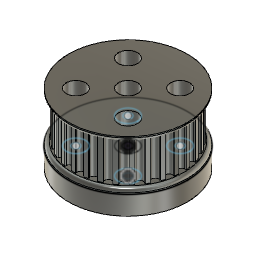
M5_Pulley_t30 v3 (Autodesk Fusion 360 design; units mm, degrees)
Autodesk Fusion 360 part; units mm, degrees
sketch "Sketch1" plane through (0, 0, 0) normal (0, 0, 1) x (1, 0, 0)
  circle A0 centre (0, 0) radius 25
  circle A1 centre (0, 0) radius 4
  circle A2 centre (0, 0) radius 1.75
  circle A3 centre (10.9602, -10.9602) radius 1.5
  circle A4 centre (10.9602, -10.9602) radius 4
  circle A5 centre (10.9602, 10.9602) radius 4
  circle A6 centre (10.9602, 10.9602) radius 1.5
  circle A7 centre (-10.9602, 10.9602) radius 4
  circle A8 centre (-10.9602, 10.9602) radius 1.5
  circle A9 centre (-10.9602, -10.9602) radius 4
  circle A10 centre (-10.9602, -10.9602) radius 1.5
  point P0 (10.9602, -10.9602)
  dimension "d1" = 50
  dimension "d2" = 8
  dimension "d3" = 3.5
  dimension "d25" = 360
  constraint coincident A0.centre A1.centre
  constraint concentric A0 A2
  constraint coincident P0 A3.centre
  measures "d1" diameter of A0
  measures "d2" diameter of A1
  measures "d3" diameter of A2
sketch "Sketch3" plane through (0, 0, 0) normal (0, 0, 1) x (1, 0, 0)
  line L0 (22.3838, 1.4892) -> (22.9524, 1.5279)
  line L1 (22.9524, -1.5279) -> (22.3838, -1.4892)
  arc A0 (22.3838, 1.4892) -> (22.3838, -1.4892) centre (22.4332, 0) ccw
  line L2 (21.585, 6.1105) -> (22.1332, 6.2666)
  arc A1 (21.585, 6.1105) -> (22.2042, 3.1972) centre (21.943, 4.6641) ccw
  line L3 (22.7685, 3.2776) -> (22.2042, 3.1972)
  line L4 (19.8429, 10.4647) -> (20.3467, 10.7314)
  arc A2 (19.8429, 10.4647) -> (21.0543, 7.7439) centre (20.4938, 9.1244) ccw
  line L5 (21.5895, 7.9398) -> (21.0543, 7.7439)
  line L6 (17.2335, 14.3616) -> (17.6709, 14.7272)
  arc A3 (17.2335, 14.3616) -> (18.9842, 11.9521) centre (18.1489, 13.1859) ccw
  line L7 (19.467, 12.255) -> (18.9842, 11.9521)
  line L8 (13.871, 17.6308) -> (14.2228, 18.0793)
  arc A4 (13.871, 17.6308) -> (16.0843, 15.6379) centre (15.0108, 16.6711) ccw
  line L9 (16.4936, 16.0347) -> (16.0843, 15.6379)
  line L10 (9.9022, 20.1295) -> (10.1531, 20.6413)
  arc A5 (9.9022, 20.1295) -> (12.4815, 18.6403) centre (11.2166, 19.4278) ccw
  line L11 (12.7994, 19.1135) -> (12.4815, 18.6403)
  line L12 (5.5007, 21.7484) -> (5.6396, 22.3012)
  arc A6 (5.5007, 21.7484) -> (8.3333, 20.828) centre (6.9323, 21.3353) ccw
  line L13 (8.5458, 21.3569) -> (8.3333, 20.828)
  line L14 (0.8587, 22.4168) -> (0.8797, 22.9864)
  arc A7 (0.8587, 22.4168) -> (3.8208, 22.1055) centre (2.3449, 22.3103) ccw
  line L15 (3.9187, 22.667) -> (3.8208, 22.1055)
  line L16 (-3.8208, 22.1055) -> (-3.9187, 22.667)
  arc A8 (-3.8208, 22.1055) -> (-0.8587, 22.4168) centre (-2.3449, 22.3103) ccw
  line L17 (-0.8797, 22.9864) -> (-0.8587, 22.4168)
  line L18 (-8.3333, 20.828) -> (-8.5458, 21.3569)
  arc A9 (-8.3333, 20.828) -> (-5.5007, 21.7484) centre (-6.9323, 21.3353) ccw
  line L19 (-5.6396, 22.3012) -> (-5.5007, 21.7484)
  line L20 (-12.4815, 18.6403) -> (-12.7994, 19.1135)
  arc A10 (-12.4815, 18.6403) -> (-9.9022, 20.1295) centre (-11.2166, 19.4278) ccw
  line L21 (-10.1531, 20.6413) -> (-9.9022, 20.1295)
  line L22 (-16.0843, 15.6379) -> (-16.4936, 16.0347)
  arc A11 (-16.0843, 15.6379) -> (-13.871, 17.6308) centre (-15.0108, 16.6711) ccw
  line L23 (-14.2228, 18.0793) -> (-13.871, 17.6308)
  line L24 (-18.9842, 11.9521) -> (-19.467, 12.255)
  arc A12 (-18.9842, 11.9521) -> (-17.2335, 14.3616) centre (-18.1489, 13.1859) ccw
  line L25 (-17.6709, 14.7272) -> (-17.2335, 14.3616)
  line L26 (-21.0543, 7.7439) -> (-21.5895, 7.9398)
  arc A13 (-21.0543, 7.7439) -> (-19.8429, 10.4647) centre (-20.4938, 9.1244) ccw
  line L27 (-20.3467, 10.7314) -> (-19.8429, 10.4647)
  line L28 (-22.2042, 3.1972) -> (-22.7685, 3.2776)
  arc A14 (-22.2042, 3.1972) -> (-21.585, 6.1105) centre (-21.943, 4.6641) ccw
  line L29 (-22.1332, 6.2666) -> (-21.585, 6.1105)
  line L30 (-22.3838, -1.4892) -> (-22.9524, -1.5279)
  arc A15 (-22.3838, -1.4892) -> (-22.3838, 1.4892) centre (-22.4332, 0) ccw
  line L31 (-22.9524, 1.5279) -> (-22.3838, 1.4892)
  line L32 (-21.585, -6.1105) -> (-22.1332, -6.2666)
  arc A16 (-21.585, -6.1105) -> (-22.2042, -3.1972) centre (-21.943, -4.6641) ccw
  line L33 (-22.7685, -3.2776) -> (-22.2042, -3.1972)
  line L34 (-19.8429, -10.4647) -> (-20.3467, -10.7314)
  arc A17 (-19.8429, -10.4647) -> (-21.0543, -7.7439) centre (-20.4938, -9.1244) ccw
  line L35 (-21.5895, -7.9398) -> (-21.0543, -7.7439)
  line L36 (-17.2335, -14.3616) -> (-17.6709, -14.7272)
  arc A18 (-17.2335, -14.3616) -> (-18.9842, -11.9521) centre (-18.1489, -13.1859) ccw
  line L37 (-19.467, -12.255) -> (-18.9842, -11.9521)
  line L38 (-13.871, -17.6308) -> (-14.2228, -18.0793)
  arc A19 (-13.871, -17.6308) -> (-16.0843, -15.6379) centre (-15.0108, -16.6711) ccw
  line L39 (-16.4936, -16.0347) -> (-16.0843, -15.6379)
  line L40 (-9.9022, -20.1295) -> (-10.1531, -20.6413)
  arc A20 (-9.9022, -20.1295) -> (-12.4815, -18.6403) centre (-11.2166, -19.4278) ccw
  line L41 (-12.7994, -19.1135) -> (-12.4815, -18.6403)
  line L42 (-5.5007, -21.7484) -> (-5.6396, -22.3012)
  arc A21 (-5.5007, -21.7484) -> (-8.3333, -20.828) centre (-6.9323, -21.3353) ccw
  line L43 (-8.5458, -21.3569) -> (-8.3333, -20.828)
  line L44 (-0.8587, -22.4168) -> (-0.8797, -22.9864)
  arc A22 (-0.8587, -22.4168) -> (-3.8208, -22.1055) centre (-2.3449, -22.3103) ccw
  line L45 (-3.9187, -22.667) -> (-3.8208, -22.1055)
  line L46 (3.8208, -22.1055) -> (3.9187, -22.667)
  arc A23 (3.8208, -22.1055) -> (0.8587, -22.4168) centre (2.3449, -22.3103) ccw
  line L47 (0.8797, -22.9864) -> (0.8587, -22.4168)
  line L48 (8.3333, -20.828) -> (8.5458, -21.3569)
  arc A24 (8.3333, -20.828) -> (5.5007, -21.7484) centre (6.9323, -21.3353) ccw
  line L49 (5.6396, -22.3012) -> (5.5007, -21.7484)
  line L50 (12.4815, -18.6403) -> (12.7994, -19.1135)
  arc A25 (12.4815, -18.6403) -> (9.9022, -20.1295) centre (11.2166, -19.4278) ccw
  line L51 (10.1531, -20.6413) -> (9.9022, -20.1295)
  line L52 (16.0843, -15.6379) -> (16.4936, -16.0347)
  arc A26 (16.0843, -15.6379) -> (13.871, -17.6308) centre (15.0108, -16.6711) ccw
  line L53 (14.2228, -18.0793) -> (13.871, -17.6308)
  line L54 (18.9842, -11.9521) -> (19.467, -12.255)
  arc A27 (18.9842, -11.9521) -> (17.2335, -14.3616) centre (18.1489, -13.1859) ccw
  line L55 (17.6709, -14.7272) -> (17.2335, -14.3616)
  line L56 (21.0543, -7.7439) -> (21.5895, -7.9398)
  arc A28 (21.0543, -7.7439) -> (19.8429, -10.4647) centre (20.4938, -9.1244) ccw
  line L57 (20.3467, -10.7314) -> (19.8429, -10.4647)
  line L58 (22.2042, -3.1972) -> (22.7685, -3.2776)
  arc A29 (22.2042, -3.1972) -> (21.585, -6.1105) centre (21.943, -4.6641) ccw
  line L59 (22.1332, -6.2666) -> (21.585, -6.1105)
  line L60 (22.9524, 1.5279) -> (22.7685, 3.2776)
  line L61 (22.1332, 6.2666) -> (21.5895, 7.9398)
  line L62 (20.3467, 10.7314) -> (19.467, 12.255)
  line L63 (17.6709, 14.7272) -> (16.4936, 16.0347)
  line L64 (14.2228, 18.0793) -> (12.7994, 19.1135)
  line L65 (10.1531, 20.6413) -> (8.5458, 21.3569)
  line L66 (5.6396, 22.3012) -> (3.9187, 22.667)
  line L67 (0.8797, 22.9864) -> (-0.8797, 22.9864)
  line L68 (-3.9187, 22.667) -> (-5.6396, 22.3012)
  line L69 (-8.5458, 21.3569) -> (-10.1531, 20.6413)
  line L70 (-12.7994, 19.1135) -> (-14.2228, 18.0793)
  line L71 (-16.4936, 16.0347) -> (-17.6709, 14.7272)
  line L72 (-19.467, 12.255) -> (-20.3467, 10.7314)
  line L73 (-21.5895, 7.9398) -> (-22.1332, 6.2666)
  line L74 (-22.7685, 3.2776) -> (-22.9524, 1.5279)
  line L75 (-22.9524, -1.5279) -> (-22.7685, -3.2776)
  line L76 (-22.1332, -6.2666) -> (-21.5895, -7.9398)
  line L77 (-20.3467, -10.7314) -> (-19.467, -12.255)
  line L78 (-17.6709, -14.7272) -> (-16.4936, -16.0347)
  line L79 (-14.2228, -18.0793) -> (-12.7994, -19.1135)
  line L80 (-10.1531, -20.6413) -> (-8.5458, -21.3569)
  line L81 (-5.6396, -22.3012) -> (-3.9187, -22.667)
  line L82 (-0.8797, -22.9864) -> (0.8797, -22.9864)
  line L83 (3.9187, -22.667) -> (5.6396, -22.3012)
  line L84 (8.5458, -21.3569) -> (10.1531, -20.6413)
  line L85 (12.7994, -19.1135) -> (14.2228, -18.0793)
  line L86 (16.4936, -16.0347) -> (17.6709, -14.7272)
  line L87 (19.467, -12.255) -> (20.3467, -10.7314)
  line L88 (21.5895, -7.9398) -> (22.1332, -6.2666)
  line L89 (22.7685, -3.2776) -> (22.9524, -1.5279)
  circle A30 centre (0, 0) radius 24.95
  point P0 (22.4332, 0)
  point P1 (22.9524, -1.5279)
  dimension "d27" = 360
  dimension "d29" = 360
  dimension "d30" = 49.9
  constraint coincident P0 A0.centre
  constraint coincident L0.start A0.start
  constraint coincident P1 L1.start
  constraint coincident L1.end A0.end
  constraint coincident A30.centre origin
  measures "d30" diameter of A30
extrude "Extrude1" add sketch "Sketch3" along normal blind 21 contours L0 L1 A0 L2 A1 L3 L4 A2 L5 L6 A3 L7 L8 A4 L9 L10 A5 L11 L12 A6 L13 L14 A7 L15 L16 A8 L17 L18 A9 L19 L20 A10 L21 L22 A11 L23 L24 A12 L25 L26 A13 L27 L28 A14 L29 L30 A15 L31 L32 A16 L33 L34 A17 L35 L36 A18 L37 L38 A19 L39 L40 A20 L41 L42 A21 L43 L44 A22 L45 L46 A23 L47 L48 A24 L49 L50 A25 L51 L52 A26 L53 L54 A27 L55 L56 A28 L57 L58 A29 L59 L60 L61 L62 L63 L64 L65 L66 L67 L68 L69 L70 L71 L72 L73 L74 L75 L76 L77 L78 L79 L80 L81 L82 L83 L84 L85 L86 L87 L88 L89
extrude "Extrude2" add sketch "Sketch3" along normal blind 2 and the other way blind 8 contours L0 L1 A0 L2 A1 L3 L4 A2 L5 L6 A3 L7 L8 A4 L9 L10 A5 L11 L12 A6 L13 L14 A7 L15 L16 A8 L17 L18 A9 L19 L20 A10 L21 L22 A11 L23 L24 A12 L25 L26 A13 L27 L28 A14 L29 L30 A15 L31 L32 A16 L33 L34 A17 L35 L36 A18 L37 L38 A19 L39 L40 A20 L41 L42 A21 L43 L44 A22 L45 L46 A23 L47 L48 A24 L49 L50 A25 L51 L52 A26 L53 L54 A27 L55 L56 A28 L57 L58 A29 L59 L60 L61 L62 L63 L64 L65 L66 L67 L68 L69 L70 L71 L72 L73 L74 L75 L76 L77 L78 L79 L80 L81 L82 L83 L84 L85 L86 L87 L88 L89 | A30
extrude "Extrude3" add sketch "Sketch3" along normal blind 21 and the other way blind -19
fillet "Fillet1" radius 1.5 2 edges at (-23.2616, -9.0223, 19) (-23.2616, -9.0223, 2)
extrude "Extrude4" cut sketch "Sketch1" along normal mid plane 42 contours A2 | A3 | A6 | A8 | A10
extrude "Extrude5" cut sketch "Sketch1" along normal blind 21 and the other way blind -3 contours A1 | A4 | A5 | A7 | A9
equation "teeth = 30"
equation "d60 = 50 mm - 0.1 mm"
named bodies: "T30"
